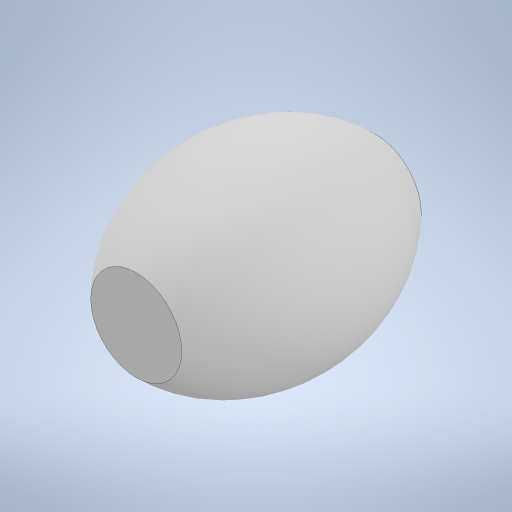
# Autodesk Inventor part: task4
Saved by Autodesk Inventor 2024.2 (Build 282272000, 272)
## iProperties
Created: 2024-10-18
Part Number: task4
Material: Типовые
Document SubType Name: Modeling
Designer: user
Density: 1 g/cm^3
Appearance: По умолчанию
Author: user
Autodesk Inventor part; units mm, degrees
ref_plane "YZ Plane" through (0, 0, 0) normal (1, 0, 0) x (0, 1, 0)
ref_plane "XZ Plane" through (0, 0, 0) normal (0, 1, 0) x (-1, 0, 0)
ref_plane "XY Plane" through (0, 0, 0) normal (0, 0, 1) x (1, 0, 0)
sketch "Эскиз1" plane through (0, 0, 0) normal (1, 0, 0) x (0, 1, 0)
  line L0 (0, 0) -> (0, -20)
  line L1 (0, -20) -> (0, 20)
  arc A0 (7.5959, -20) -> (7.5959, 20) centre (-12, 0) ccw
  line L2 (0, 20) -> (7.5959, 20)
  line L3 (0, -20) -> (7.5959, -20)
  constraints: 8 end point, 2 horizontal, 2 point on circle, 1 centre point, 1 coincident, 1 point on line, 1 vertical
revolve "Вращение1" add sketch "Эскиз1" angle 360 about axis through (0, 0, -20) along (0, 0, 1)
